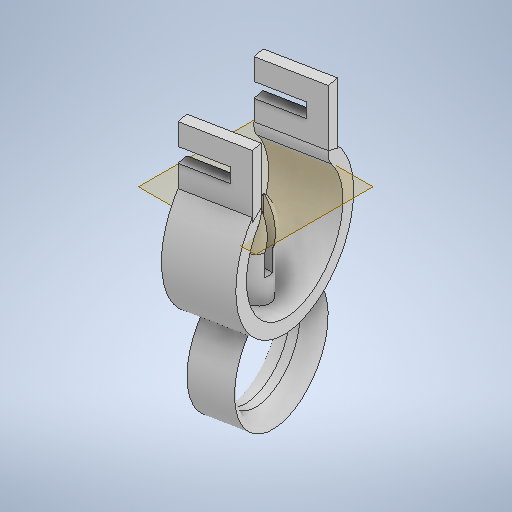
# Autodesk Inventor part: Clip3
Saved by Autodesk Inventor 2025 (Build 290162010, 162A)
## iProperties
Created: 2026-02-19
Part Number: Clip3
Material: Generic
Document SubType Name: Modeling
Designer: 925699
Density: 1 g/cm^3
Appearance: Default
Author: 925699
Autodesk Inventor part; units mm, degrees
ref_plane "YZ Plane" through (0, 0, 0) normal (1, 0, 0) x (0, 1, 0)
sketch "Sketch1" plane through (0, 0, 0) normal (0, 0, 1) x (1, 0, 0)
  line L0 (0, 0) -> (2.54, 0)
  line L1 (2.54, 0) -> (2.54, 8.6967)
  line L2 (0, 0) -> (0, 17.8837)
  arc A0 (2.54, 8.6967) -> (0, 17.8837) centre (-5.1799, 11.5069) ccw
  dimension "d0" = 2.54
  constraints: 6 end point, 2 point on circle, 1 centre point, 1 horizontal, 1 vertical
  measures "d0" distance of L0.start L0.end
ref_plane "Work Plane3" through (0, 17.8837, 0) normal (0, 1, 0) x (1, 0, 0)
ref_plane "Work Plane1" through (-3.9896, 4.3483, 0.7741) normal (-0.9816919, 0, 0.1904757) x (0, -1, 0)
sketch "Sketch3" plane through (-3.9896, 4.3483, 0.7741) normal (-0.9816919, 0, 0.1904757) x (0, -1, 0)
  arc A0 (-16.337, -6.8791) -> (-16.337, 6.8791) centre (-7.2089, 0) ccw
  arc A1 (-18.3655, -8.4078) -> (-18.3655, 8.4078) centre (-7.2089, 0) ccw
  line L0 (-13.5354, -0.5887) -> (0.7521, -0.5887) projected
  line L1 (-13.5354, 0.6171) -> (0.7521, 0.6171) projected
  line L2 (-7.2089, 0) -> (-7.9901, -0.5887)
  line L3 (-16.337, -6.8791) -> (-18.3655, -8.4078)
  line L4 (-7.2089, 0) -> (-8.0277, 0.6171)
  line L5 (-16.337, 6.8791) -> (-18.3655, 8.4078)
  constraints: 8 end point, 4 point on circle, 2 centre point, 2 coincident, 2 point on line
extrude "Extrusion2" add sketch "Sketch3" along normal blind 1.5875 and the other way blind 10.3124
fillet "Fillet1" radius 3.175 2 edges at (-1.0173, 20.6854, -6.81) (1.6033, 20.6854, 6.6963)
ref_plane "Work Plane2" through (0.293, 4.3483, -0.0568) normal (0.9816919, 0, -0.1904757) x (-0.1904757, 0, -0.9816919)
sketch "Sketch4" plane through (0.293, 4.3483, -0.0568) normal (0.9816919, 0, -0.1904757) x (-0.1904757, 0, -0.9816919)
  circle A0 centre (0, -12.1867) radius 8.89
  arc A1 (-8.4078, 18.3655) -> (8.4078, 18.3655) centre (0, 7.2089) ccw projected
  arc A2 (-7.848, -4.3483) -> (7.848, -4.3483) centre (0, -12.1867) ccw
  point P0 (0, -4.3483)
  point P1 (5.8384, -5.4826)
  point P2 (-5.8384, -5.4826)
  dimension "d17" = 17.78
  constraints: 4 point on circle, 2 centre point, 1 concentric
  measures "d17" diameter of A0
extrude "Extrusion3" add sketch "Sketch4" along normal mid plane 7.62 contours A0 A1 A2
fillet "Fillet2" radius 3.175 2 edges at (-3.4473, -16.7283, 0.6689) (4.0332, -16.7283, -0.7826)
sketch "Sketch5" plane through (-5.548, 4.3483, 1.0765) normal (-0.9816919, 0, 0.1904757) x (0.1904757, 0, 0.9816919)
  arc A0 (-8.6921, 14.6313) -> (-8.4078, 18.3655) centre (-11.1066, 16.6931) ccw projected
  line L0 (-7.9735, 17.2071) -> (-7.9735, 24.0368)
  line L1 (-10.116, 24.0368) -> (-10.116, 16.3667)
  arc A1 (8.4078, 18.3655) -> (8.6921, 14.6313) centre (11.1066, 16.6931) ccw projected
  line L2 (7.9735, 17.2071) -> (7.9735, 24.0368)
  line L3 (10.0556, 24.0368) -> (10.0556, 16.0648)
  line L4 (-10.116, 16.3667) -> (-7.9735, 17.2071)
  line L5 (7.9735, 17.2071) -> (10.0556, 16.0648)
  line L6 (10.0556, 24.0368) -> (10.0556, 27.7976)
  line L7 (7.9735, 27.7976) -> (7.9735, 21.3706)
  line L8 (-7.9735, 24.0368) -> (-7.9735, 27.7976)
  line L9 (-10.116, 27.7976) -> (-10.116, 24.0368)
  line L10 (-10.116, 27.7976) -> (-7.9735, 27.7976)
  line L11 (7.9735, 27.7976) -> (10.0556, 27.7976)
  point P0 (0, -4.3483)
  point P1 (-7.9735, 31.5584)
  point P2 (-10.116, 31.5584)
  constraints: 24 end point, 3 vertical, 2 point on circle, 2 point on line, 1 parallel
extrude "Extrusion4" add sketch "Sketch5" against normal blind 11.9126
sketch "Sketch6" plane through (-5.548, 4.3483, 1.0765) normal (-0.9816919, 0, 0.1904757) x (0.1904757, 0, 0.9816919)
  line L0 (11.5164, 23.7535) -> (-13.6635, 23.7535)
  line L1 (-13.6635, 23.7535) -> (-13.6635, 21.0208)
  line L2 (-13.6635, 21.0208) -> (11.5164, 21.0208)
  line L3 (11.5164, 21.0208) -> (11.5164, 23.7535)
  point P0 (0, -4.3483)
  constraints: 8 end point, 2 parallel, 1 horizontal, 1 perpendicular
extrude "Extrusion5" cut sketch "Sketch6" against normal blind 8.382
revolve "Revolution2" add sketch "Sketch1" angle 360 about axis through (0, 0, 0) along (0, 1, 0)
sketch "Sketch7" plane through (0, 17.8837, 0) normal (0, 1, 0) x (1, 0, 0)
  line L0 (0.762, -4.5728) -> (-0.762, -4.5728)
  line L1 (-0.762, -4.5728) -> (-0.762, 4.195)
  line L2 (-0.762, 4.195) -> (0.762, 4.195)
  line L3 (0.762, 4.195) -> (0.762, -4.5728)
  line L4 (4.5728, 0.762) -> (4.5728, -0.762)
  line L5 (4.5728, -0.762) -> (-4.195, -0.762)
  line L6 (-4.195, -0.762) -> (-4.195, 0.762)
  line L7 (-4.195, 0.762) -> (4.5728, 0.762)
  point P0 (0, 0)
  point P1 (-0.762, -0.762)
  point P2 (0.762, -0.762)
  point P3 (0.762, 0.762)
  point P4 (-0.762, 0.762)
  dimension "d30" = 90
  dimension "d34" = 0.762
  dimension "d35" = 0.762
  constraints: 16 end point, 2 parallel, 1 horizontal, 1 perpendicular, 9 other
  measures "d34" distance from line of point (0, 0) L7
  measures "d35" distance from line of point (0, 0) L5
extrude "Extrusion6" cut sketch "Sketch7" against normal blind 13.1445
body "Solid1"
